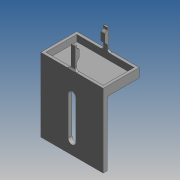
# Autodesk Inventor part: P036_SupportLidar
Saved by Autodesk Inventor 2021.3 (Build 253353000, 353)
## iProperties
Created: 2021-11-26
Part Number: P036_SupportLidar
Material: Générique
Document SubType Name: Modeling
Designer: gabri
Density: 1 g/cm^3
Appearance: Par défaut
Author: gabri
Autodesk Inventor part; units mm, degrees
ref_plane "YZ Plane" through (0, 0, 0) normal (1, 0, 0) x (0, 1, 0)
ref_plane "XZ Plane" through (0, 0, 0) normal (0, 1, 0) x (-1, 0, 0)
ref_plane "XY Plane" through (0, 0, 0) normal (0, 0, 1) x (1, 0, 0)
sketch "Sketch2" plane through (0, 0, 0) normal (0, 0, 1) x (1, 0, 0)
  line L0 (22.25, 12) -> (-22.25, 12)
  line L1 (-22.25, 12) -> (-22.25, -12)
  line L2 (-22.25, -12) -> (22.25, -12)
  line L3 (22.25, -12) -> (22.25, 12)
  line L4 (22.25, 12) -> (-22.25, -12) construction
  line L5 (-22.25, 12) -> (22.25, -12) construction
  line L6 (24.25, 14) -> (-24.25, 14)
  line L7 (-24.25, 14) -> (-24.25, -14)
  line L8 (-24.25, -14) -> (24.25, -14)
  line L9 (24.25, -14) -> (24.25, 14)
  line L10 (24.25, 14) -> (-24.25, -14) construction
  line L11 (-24.25, 14) -> (24.25, -14) construction
  point P0 (0, 0)
  dimension "d0" = 44.5
  dimension "d1" = 24
  dimension "d2" = 48.5
  dimension "d3" = 28
  constraints: 24 end point, 4 midpoint, 4 parallel, 2 horizontal, 2 perpendicular
  measures "d0" distance of L2.end L1.end
  measures "d1" distance between parallel lines of L0 L2
  measures "d2" distance of L7.end L8.end
  measures "d3" distance between parallel lines of L6 L8
extrude "Extrusion1" add sketch "Sketch2" along normal blind 5
sketch "Sketch3" plane through (0, 0, 5) normal (0, 0, 1) x (1, 0, 0)
  line L0 (-24.25, 14) -> (-24.25, -14) construction
  line L1 (-24.25, -14) -> (24.25, -14) construction
  line L2 (24.25, -14) -> (24.25, 14) construction
  line L3 (24.25, 14) -> (-24.25, 14) construction
  line L4 (22.25, 12) -> (22.25, -12) construction
  line L5 (22.25, -12) -> (-22.25, -12) construction
  line L6 (-22.25, -12) -> (-22.25, 12) construction
  line L7 (-22.25, 12) -> (22.25, 12) construction
  line L8 (1.5, -13) -> (-1.5, -13)
  line L9 (-1.5, -13) -> (-1.5, -12)
  line L10 (-1.5, -12) -> (1.5, -12)
  line L11 (1.5, -12) -> (1.5, -13)
  line L12 (1.5, -13) -> (-1.5, -12) construction
  line L13 (-1.5, -13) -> (1.5, -12) construction
  line L14 (1.5, 13) -> (-1.5, 13)
  line L15 (-1.5, 13) -> (-1.5, 12)
  line L16 (-1.5, 12) -> (1.5, 12)
  line L17 (1.5, 12) -> (1.5, 13)
  line L18 (1.5, 13) -> (-1.5, 12) construction
  line L19 (-1.5, 13) -> (1.5, 12) construction
  line L20 (0, 19.6) -> (0, -19.6) construction
  point P0 (0, 0)
  point P1 (0, -12.5)
  point P2 (0, -12.5)
  point P3 (0, 12.5)
  point P4 (0, 12.5)
  dimension "d8" = 3
  dimension "d19" = 1
  dimension "d22" = 3
  dimension "d23" = 1
  constraints: 24 end point, 6 midpoint, 4 parallel, 3 point on line, 2 horizontal, 2 perpendicular
  measures "d8" distance between parallel lines of L11 L9
  measures "d19" distance between parallel lines of L10 L8
  measures "d22" distance of L14.start L14.end
  measures "d23" distance between parallel lines of L14 L16
extrude "Extrusion2" add sketch "Sketch3" along normal blind 16.5
sketch "Sketch4" plane through (-22.25, -12, 0) normal (0, 1, 0) x (1, 0, 0)
  line L0 (44.5, 0) -> (0, 0) construction
  line L1 (0, 0) -> (0, -5) construction
  line L2 (20.75, -5) -> (0, -5) construction
  line L3 (20.75, -5) -> (20.75, -21.5) construction
  line L4 (23.75, -21.5) -> (20.75, -21.5) construction
  line L5 (23.75, -5) -> (23.75, -21.5) construction
  line L6 (44.5, -5) -> (23.75, -5) construction
  line L7 (44.5, 0) -> (44.5, -5) construction
  line L8 (20.75, -19) -> (23.75, -19)
  line L9 (23.75, -19) -> (23.75, -10)
  line L10 (23.75, -10) -> (20.75, -10)
  line L11 (20.75, -10) -> (20.75, -19)
  line L12 (20.75, -19) -> (23.75, -10) construction
  line L13 (23.75, -19) -> (20.75, -10) construction
  line L14 (22.25, 4.3) -> (22.25, -25.8) construction
  point P0 (22.25, 0)
  point P1 (22.25, -14.5)
  point P2 (22.25, -14.5)
  dimension "d12" = 10
  dimension "d13" = 9
  constraints: 12 end point, 3 midpoint, 2 parallel, 2 point on line, 1 horizontal, 1 perpendicular
  measures "d12" distance between parallel lines of L0 L10
  measures "d13" distance between parallel lines of L10 L8
extrude "Extrusion3" add sketch "Sketch4" along normal blind 2
sketch "Sketch5" plane through (1.5, -14, 5) normal (1, 0, 0) x (0, 0, -1)
  line L0 (0, 2) -> (0, 1) construction
  line L1 (0, 2) -> (-5, 2) construction
  line L2 (-5, 2) -> (-5, 4) construction
  line L3 (-14, 4) -> (-5, 4) construction
  line L4 (-14, 2) -> (-14, 4) construction
  line L5 (-14, 2) -> (-16.5, 2) construction
  line L6 (-16.5, 1) -> (-16.5, 2) construction
  line L7 (0, 1) -> (-16.5, 1) construction
  line L8 (-5, 2) -> (-7, 4)
  line L9 (-5, 2) -> (-5, 4)
  line L10 (-7, 4) -> (-5, 4)
  point P0 (5, 14)
  dimension "d16" = 2
  constraints: 6 end point, 2 collinear, 1 point on line
  measures "d16" horizontal distance of L8.end L1.end
extrude "Extrusion4" cut sketch "Sketch5" against normal up to surface (3 mm away)
sketch "Sketch6" plane through (-22.25, 12, 0) normal (0, -1, 0) x (1, 0, 0)
  line L0 (23.75, 12) -> (20.75, 12) construction
  line L1 (20.75, 10) -> (23.75, 10) construction
  line L2 (23.75, 19) -> (20.75, 19) construction
  line L3 (20.75, 19) -> (23.75, 19)
  line L4 (23.75, 19) -> (23.75, 10)
  line L5 (23.75, 10) -> (20.75, 10)
  line L6 (20.75, 10) -> (20.75, 19)
  point P0 (22.25, 0)
  constraints: 8 end point, 2 parallel, 1 horizontal, 1 perpendicular
extrude "Extrusion5" add sketch "Sketch6" along normal blind 2
sketch "Sketch8" plane through (1.5, 12, 5) normal (1, 0, 0) x (0, 0, -1)
  line L0 (0, 1) -> (0, 0) construction
  line L1 (0, 1) -> (-16.5, 1) construction
  line L2 (-16.5, 0) -> (-16.5, 1) construction
  line L3 (-14, 0) -> (-16.5, 0) construction
  line L4 (-14, 0) -> (-14, -2) construction
  line L5 (-5, -2) -> (-14, -2) construction
  line L6 (-5, 0) -> (-5, -2) construction
  line L7 (0, 0) -> (-5, 0) construction
  line L8 (-7, -2) -> (-5, 0)
  line L9 (-7, -2) -> (-5, -2)
  line L10 (-5, -2) -> (-5, 0)
  point P0 (5, -12)
  dimension "d26" = 2
  constraints: 6 end point, 1 collinear, 1 point on line
  measures "d26" distance of L5.start L8.start
extrude "Extrusion6" cut sketch "Sketch8" against normal up to surface (3 mm away)
fillet "Fillet1" radius 2 6 edges at (1.5, -12.5, 5) (0, -13, 5) (-1.5, -12.5, 5) (1.5, 12.5, 5) (0, 13, 5) (-1.5, 12.5, 5)
fillet "Fillet2" radius 1 4 edges at (0, -12, 10) (0, -10, 12) (0, 12, 10) (0, 10, 12)
sketch "Sketch9" plane through (0, 0, 0) normal (0, 0, -1) x (-1, 0, 0)
  line L0 (24.25, 14) -> (24.25, -14) construction
  line L1 (-24.25, 14) -> (24.25, 14) construction
  line L2 (-24.25, -14) -> (-24.25, 14) construction
  line L3 (24.25, -14) -> (-24.25, -14) construction
  line L4 (-22.25, 12) -> (-22.25, -12) construction
  line L5 (22.25, 12) -> (-22.25, 12) construction
  line L6 (22.25, -12) -> (22.25, 12) construction
  line L7 (-22.25, -12) -> (22.25, -12) construction
  line L8 (-24.25, 14) -> (24.25, 14)
  line L9 (24.25, 14) -> (24.25, -14)
  line L10 (24.25, -14) -> (-24.25, -14)
  line L11 (-24.25, -14) -> (-24.25, 14)
  point P0 (0, 0)
  constraints: 8 end point, 2 parallel, 1 horizontal, 1 perpendicular
extrude "Extrusion7" add sketch "Sketch9" along normal blind 2
fillet "Fillet3" radius 1 2 edges at (0, -12, 19) (0, 12, 19)
fillet "Fillet4" radius 1 2 edges at (0, -10, 19) (0, 10, 19)
sketch "Sketch10" plane through (0, 0, -2) normal (0, 0, -1) x (-1, 0, 0)
  line L0 (-22.25, -12) -> (22.25, -12) construction
  line L1 (-24.25, -14) -> (24.25, -14) construction
  line L2 (24.25, -14) -> (24.25, 14) construction
  line L3 (24.25, 14) -> (-24.25, 14) construction
  line L4 (-24.25, 14) -> (-24.25, -14) construction
  line L5 (-24.25, -14) -> (24.25, -14)
  line L6 (24.25, -14) -> (24.25, -11)
  line L7 (24.25, -11) -> (-24.25, -11)
  line L8 (-24.25, -11) -> (-24.25, -14)
  point P0 (0, 0)
  dimension "d35" = 3
  constraints: 8 end point, 2 parallel, 1 horizontal, 1 perpendicular, 1 point on line
  measures "d35" distance between parallel lines of L1 L7
extrude "Extrusion8" add sketch "Sketch10" along normal blind 50
sketch "Sketch11" plane through (3.5, -14, 5) normal (0, -1, 0) x (1, 0, 0)
  line L0 (20.75, -7) -> (-27.75, -7) construction
  line L1 (-3.5, -47) -> (-3.5, -17) construction
  line L2 (-0.5, -47) -> (-0.5, -17)
  line L3 (-6.5, -17) -> (-6.5, -47)
  arc A0 (-6.5, -47) -> (-0.5, -47) centre (-3.5, -47) ccw
  arc A1 (-0.5, -17) -> (-6.5, -17) centre (-3.5, -17) ccw
  line L4 (20.75, -57) -> (-27.75, -57) construction
  line L5 (-3.5, 31.2) -> (-3.5, -71.7) construction
  point P0 (-3.5, -5)
  point P1 (-3.5, -32)
  dimension "d38" = 6
  dimension "d39" = 25
  dimension "d40" = 25
  dimension "d41" = 30
  dimension "d42" = 3
  constraints: 8 end point, 4 point on circle, 4 tangent, 2 centre point, 1 midpoint, 1 parallel, 1 point on line, 1 vertical
  measures "d38" diameter of A1
  measures "d39" distance from line of L4 point (-3.5, -32)
  measures "d40" distance from line of L0 point (-3.5, -32)
  measures "d41" distance of L2.start L2.end
  measures "d42" radius of A0
extrude "Extrusion9" cut sketch "Sketch11" against normal blind 10
fillet "Fillet5" radius 2 1 edges at (0, -11, -2)
body "Solid1"
